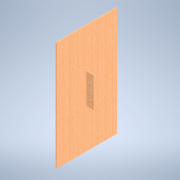
# Autodesk Inventor part: rightside
Saved by Autodesk Inventor 2020 (Build 240168000, 168)
## iProperties
Created: 2020-05-02
Part Number: rightside
Material: Generic
Document SubType Name: Modeling
Designer: galaxy
Density: 1 g/cm^3
Appearance: Default
Author: galaxy
Autodesk Inventor part; units mm, degrees
ref_plane "YZ Plane" through (0, 0, 0) normal (1, 0, 0) x (0, 1, 0)
ref_plane "XZ Plane" through (0, 0, 0) normal (0, 1, 0) x (-1, 0, 0)
ref_plane "XY Plane" through (0, 0, 0) normal (0, 0, 1) x (1, 0, 0)
sketch "Sketch1" plane through (0, 0, 0) normal (1, 0, 0) x (0, 1, 0)
  line L0 (180, 100) -> (-180, 100)
  line L1 (-180, 100) -> (-180, -100)
  line L2 (-180, -100) -> (180, -100)
  line L3 (180, -100) -> (180, 100)
  line L4 (180, 100) -> (-180, -100) construction
  line L5 (-180, 100) -> (180, -100) construction
  point P0 (0, 0)
  dimension "d0" = 360
  dimension "d1" = 200
  constraints: 12 end point, 2 midpoint, 2 parallel, 1 horizontal, 1 perpendicular
  measures "d0" distance of L2.end L1.end
  measures "d1" distance of L1.end L0.end
extrude "Extrusion1" add sketch "Sketch1" along normal blind 3
sketch "Sketch7" plane through (3, 0, 0) normal (1, 0, 0) x (0, 0, -1)
  line L0 (1.5, 50) -> (-1.5, 50)
  line L1 (-1.5, 50) -> (-1.5, -50)
  line L2 (-1.5, -50) -> (1.5, -50)
  line L3 (1.5, -50) -> (1.5, 50)
  line L4 (1.5, 50) -> (-1.5, -50) construction
  line L5 (-1.5, 50) -> (1.5, -50) construction
  point P0 (0, 0)
  dimension "d69" = 3
  dimension "d70" = 100
  constraints: 12 end point, 2 midpoint, 2 parallel, 1 horizontal, 1 perpendicular
  measures "d69" distance of L2.end L1.end
  measures "d70" distance of L1.end L0.end
extrude "Extrusion10" add sketch "Sketch7" along normal blind 24
sketch "Sketch8" plane through (3, -50, 1.5) normal (0, 0, 1) x (1, 0, 0)
  circle A0 centre (13, 75) radius 1.5
  circle A1 centre (13, 50) radius 1.5
  circle A2 centre (13, 25) radius 1.5
  line L0 (0, 100) -> (24, 100) projected
  line L1 (0, 0) -> (24, 0) projected
  line L2 (24, 100) -> (24, 0) projected
  line L3 (0, 230) -> (0, -130) projected
  point P0 (-3, 50)
  dimension "d73" = 3
  dimension "d74" = 3
  dimension "d75" = 3
  dimension "d76" = 25
  dimension "d77" = 25
  dimension "d78" = 25
  dimension "d87" = 25
  dimension "d88" = 11
  dimension "d89" = 11
  dimension "d90" = 11
  constraints: 3 centre point
  measures "d73" diameter of A0
  measures "d74" diameter of A1
  measures "d75" diameter of A2
  measures "d76" distance from line of L0 A0.centre
  measures "d77" distance from line of A2.centre L1
  measures "d78" distance of A0.centre A1.centre
  measures "d87" distance of A1.centre A2.centre
  measures "d88" distance from line of L2 A0.centre
  measures "d89" distance from line of L2 A1.centre
  measures "d90" distance from line of L2 A2.centre
extrude "Extrusion11" cut sketch "Sketch8" against normal blind 25 contours A0 | A1 | A2
body "Solid1"
